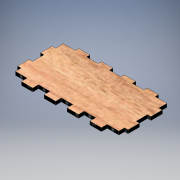
# Autodesk Inventor part: TopBottomPlate
Saved by Autodesk Inventor 2019.4 (Build 234330000, 330)
## iProperties
Created: 2020-06-30
Part Number: TopBottomPlate
Material: Wood (Birch)
Document SubType Name: Modeling
Designer: wimva
Density: 0.55 g/cm^3
Appearance: Birch - Natural Polished
Author: wimva
Autodesk Inventor part; units mm, degrees
ref_plane "YZ Plane" through (0, 0, 0) normal (1, 0, 0) x (0, 1, 0)
ref_plane "XZ Plane" through (0, 0, 0) normal (0, 1, 0) x (-1, 0, 0)
ref_plane "XY Plane" through (0, 0, 0) normal (0, 0, 1) x (1, 0, 0)
sketch "Sketch1" plane through (0, 0, 0) normal (0, 1, 0) x (-1, 0, 0)
  line L0 (-48.26, 25) -> (48.26, 25)
  line L1 (48.26, 25) -> (48.26, -25)
  line L2 (48.26, -25) -> (-48.26, -25)
  line L3 (-48.26, -25) -> (-48.26, 25)
  line L4 (-48.26, 25) -> (48.26, -25) construction
  line L5 (48.26, 25) -> (-48.26, -25) construction
  point P0 (0, 0)
  dimension "d0" = 96.52
  dimension "d1" = 50
  constraints: 12 end point, 2 midpoint, 2 parallel, 1 horizontal, 1 perpendicular
  measures "d0" distance of L1.end L2.end
  measures "d1" distance of L0.end L1.end
extrude "Extrusion1" add sketch "Sketch1" along normal blind 3
sketch "Sketch2" plane through (0, 3, 0) normal (0, 1, 0) x (1, 0, 0)
  line L0 (48.26, 25) -> (-48.26, 25) construction
  line L1 (-5, 25) -> (5, 25)
  line L2 (5, 25) -> (5, 22)
  line L3 (5, 22) -> (-5, 22)
  line L4 (-5, 22) -> (-5, 25)
  line L5 (0, 35) -> (0, -35) construction
  point P0 (0, 0)
  dimension "d4" = 10
  dimension "d5" = 3
  constraints: 8 end point, 2 parallel, 1 horizontal, 1 perpendicular, 1 point on line, 1 other
  measures "d4" distance of L2.end L3.end
  measures "d5" distance of L1.end L2.end
extrude "Extrusion2" cut sketch "Sketch2" against normal blind 3
pattern_linear "Rectangular Pattern1" count 3 spacing 20 along (-1, 0, 0) count 2 spacing 40 along (1, 0, 0) of "Extrusion2"
sketch "Sketch3" plane through (0, 3, 0) normal (0, 1, 0) x (1, 0, 0)
  line L0 (-48.26, -25) -> (48.26, -25) construction
  line L1 (-5, -25) -> (5, -25)
  line L2 (5, -25) -> (5, -20)
  line L3 (5, -20) -> (-5, -20)
  line L4 (-5, -20) -> (-5, -25)
  line L5 (0, 35) -> (0, -35) construction
  point P0 (0, 0)
  dimension "d14" = 10
  dimension "d15" = 5
  constraints: 8 end point, 2 parallel, 1 horizontal, 1 perpendicular, 1 point on line, 1 other
  measures "d14" distance of L2.end L3.end
  measures "d15" distance of L1.end L2.end
extrude "Extrusion3" cut sketch "Sketch3" against normal through all
pattern_linear "Rectangular Pattern2" count 3 spacing 20 along (-1, 0, 0) count 2 spacing 40 along (1, 0, 0) of "Extrusion3"
sketch "Sketch4" plane through (0, 3, 0) normal (0, 1, 0) x (1, 0, 0)
  line L0 (-48.26, 25) -> (-48.26, -25) construction
  line L1 (-48.26, -25) -> (-48.26, 25) construction
  line L2 (-48.26, 5) -> (-45.26, 5)
  line L3 (-45.26, 5) -> (-45.26, -5)
  line L4 (-45.26, -5) -> (-48.26, -5)
  line L5 (-48.26, -5) -> (-48.26, 5)
  line L6 (67.564, 0) -> (-67.564, 0) construction
  point P0 (0, 0)
  dimension "d24" = 3
  dimension "d25" = 10
  constraints: 8 end point, 2 parallel, 1 horizontal, 1 perpendicular, 1 point on line, 1 other
  measures "d24" distance of L3.end L4.end
  measures "d25" distance of L2.end L3.end
extrude "Extrusion4" cut sketch "Sketch4" against normal through all
pattern_linear "Rectangular Pattern3" count 2 spacing 20 along (0, 0, -1) count 2 spacing 40 along (0, 0, 1) of "Extrusion4"
mirror "Mirror1" about plane through (0, 0, 0) normal (1, 0, 0) of "Extrusion4", "Rectangular Pattern3"
sketch "Sketch5" plane through (0, 3, 0) normal (0, 1, 0) x (1, 0, 0)
  line L0 (-45, 22) -> (-35, 22) construction
  line L1 (-45.26, 25) -> (-45.26, 15) construction
  line L2 (-45, 22) -> (-45.26, 22)
  line L3 (-45.26, 22) -> (-45.26, 25)
  line L4 (-45.26, 25) -> (-45, 25)
  line L5 (-45, 25) -> (-45, 22)
  line L6 (-45, -25) -> (-45, -20) projected
  line L7 (-45.26, -25) -> (-45, -25) projected
  line L8 (-45, -20) -> (-45.26, -20)
  line L9 (-45.26, -20) -> (-45.26, -25)
  line L10 (-45.26, -25) -> (-45, -25)
  line L11 (-45, -25) -> (-45, -20)
  point P0 (0, 0)
  constraints: 16 end point, 4 parallel, 2 horizontal, 2 perpendicular
extrude "Extrusion5" cut sketch "Sketch5" against normal through all
mirror "Mirror2" about plane through (0, 0, 0) normal (1, 0, 0) of "Extrusion5"
equation "\"d0\" = Module_Width"
equation "\"d1\" = Module_Depth"
equation "\"d2\" = Module_Case_Thickness"
equation "\"d4\" = Module_Case_SlotWidth"
equation "\"d5\" = Module_Case_SlotDepth"
equation "\"d6\" = Module_Case_Thickness"
equation "\"d10\" = 2 * Module_Case_SlotWidth"
equation "\"d13\" = 4 * Module_Case_SlotWidth"
equation "\"d14\" = Module_Case_SlotWidth"
equation "\"d15\" = Module_Case_BottomSlotDepth"
equation "\"d16\" = Module_Case_Thickness"
equation "\"d20\" = 2 * Module_Case_SlotWidth"
equation "\"d23\" = 4 * Module_Case_SlotWidth"
equation "\"d24\" = Module_Case_SlotDepth"
equation "\"d25\" = Module_Case_SlotWidth"
equation "\"d26\" = Module_Case_Thickness"
equation "\"d30\" = 2 * Module_Case_SlotWidth"
equation "\"d33\" = 4 * Module_Case_SlotWidth"
equation "\"RackWidth\" = 482.6"
equation "\"U\" = 44.5"
equation "\"Module_Width\" = 96.52"
equation "\"Module_Height\" = 89"
equation "\"Module_Depth\" = 50"
equation "\"Module_Case_Thickness\" = 3"
equation "\"Module_Back_Thickness\" = 5"
equation "\"Module_Case_SlotDepth\" = 3"
equation "\"Module_Case_BottomSlotDepth\" = 5"
equation "\"Module_Case_SlotWidth\" = 10"
equation "\"Module_Connector_Width\" = 6"
equation "\"Module_Connector_Depth\" = 4"
equation "\"Module_StatusIndicatorDiameter\" = 5"
body "Solid1"
